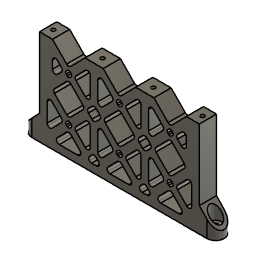
platform_hangfa-discovery-q2_top-plate-support-basic (Autodesk Fusion 360 design; units mm, degrees)
Autodesk Fusion 360 part; units mm, degrees
sketch "Sketch1" plane through (0, 0, 0) normal (0, 1, 0) x (1, 0, 0)
  circle A0 centre (0, 0) radius 2.25
  circle A1 centre (0, 0) radius 6
  circle A2 centre (0, 0) radius 9
  circle A3 centre (183.5, 0) radius 2.25
  circle A4 centre (183.5, 0) radius 6
  circle A5 centre (183.5, 0) radius 9
  line L0 (0, 0) -> (183.5, 0)
  line L1 (0, -9) -> (183.5, -9)
  line L2 (0, 9) -> (183.5, 9)
  line L3 (91.75, 9) -> (91.75, -9)
  line L4 (8, 9) -> (175.5, 9)
  line L5 (175.5, 9) -> (175.5, -9)
  line L6 (175.5, -9) -> (8, -9)
  line L7 (8, -9) -> (8, 9)
  line L8 (8, 9) -> (175.5, -9) construction
  line L9 (175.5, 9) -> (8, -9) construction
  line L10 (8, 9) -> (16, 9)
  line L11 (16, 9) -> (16, -9)
  line L12 (16, -9) -> (8, -9)
  line L13 (8, -9) -> (8, 9)
  line L14 (61.1667, -9) -> (61.1667, 9)
  line L15 (61.1667, 9) -> (69.1667, 9)
  line L16 (69.1667, 9) -> (69.1667, -9)
  line L17 (69.1667, -9) -> (61.1667, -9)
  line L18 (114.3333, -9) -> (114.3333, 9)
  line L19 (114.3333, 9) -> (122.3333, 9)
  line L20 (122.3333, 9) -> (122.3333, -9)
  line L21 (122.3333, -9) -> (114.3333, -9)
  line L22 (167.5, -9) -> (167.5, 9)
  line L23 (167.5, 9) -> (175.5, 9)
  line L24 (175.5, 9) -> (175.5, -9)
  line L25 (175.5, -9) -> (167.5, -9)
  point P0 (183.5, 0)
  point P1 (91.75, 0)
  dimension "d1" = 4.5
  dimension "d2" = 12
  dimension "d3" = 18
  dimension "d6" = 183.5
  dimension "d7" = 0
  dimension "d11" = 9
  dimension "d12" = -9
  dimension "d16" = 167.5
  dimension "d17" = 18
  dimension "d18" = 8
  dimension "d19" = 18
  dimension "d22" = 159.5
  dimension "d23" = 0
  constraint coincident A0.centre A1.centre
  constraint concentric A0 A1
  constraint coincident P0 A3.centre
  constraint midpoint L2 L3.start
  constraint midpoint L1 L3.end
  constraint perpendicular L1 L3
  constraint horizontal L4
  constraint perpendicular L4 L5
  constraint parallel L4 L6
  constraint parallel L5 L7
  constraint coincident L8 P1
  constraint coincident L9 P1
  constraint midpoint L3 P1
  constraint horizontal L10
  constraint vertical L11
  constraint horizontal L12
  constraint vertical L13
  measures "d1" diameter of A0
  measures "d2" diameter of A1
  measures "d3" diameter of A2
  measures "d16" distance of L5.end L6.end
  measures "d17" distance of L4.end L5.end
  measures "d18" distance of L4.start L10.end
  measures "d19" distance of L4.start L6.end
extrude "Extrude1" add sketch "Sketch1" against normal blind 8 contours A1 | A2 L7 L13 | A2 L2 L7 L13 | A2 L1 L7 L13 | A2 L0 L2 L4 L7 L10 L11 L13 | A2 L0 L7 L13 | A2 L0 L7 L13 | A2 L0 L1 L6 L7 L11 L12 L13 | L0 L2 L4 L11 L14 | L0 L1 L6 L11 L14 | L0 L2 L4 L14 L15 L16 | L0 L1 L6 L14 L16 L17 | L0 L2 L3 L4 L16 | L0 L1 L3 L6 L16 | L0 L2 L3 L4 L18 | L0 L1 L3 L6 L18 | L0 L2 L4 L18 L19 L20 | L0 L1 L6 L18 L20 L21 | L0 L2 L4 L20 L22 | L0 L1 L6 L20 L22 | A5 L0 L2 L4 L5 L22 L23 L24 | A5 L0 L1 L5 L6 L22 L24 L25 | A5 L2 L5 L24 | A5 L1 L5 L24 | A5 L0 L5 L24 | A5 L0 L5 L24 | A5 L5 L24 | A4
extrude "Extrude2" add sketch "Sketch1" along normal blind 92 contours A2 L0 L2 L4 L7 L10 L11 L13 | A2 L0 L7 L13 | A2 L0 L7 L13 | A2 L0 L1 L6 L7 L11 L12 L13 | L0 L2 L4 L14 L15 L16 | L0 L1 L6 L14 L16 L17 | L0 L2 L4 L18 L19 L20 | L0 L1 L6 L18 L20 L21 | A5 L0 L2 L4 L5 L22 L23 L24 | A5 L0 L1 L5 L6 L22 L24 L25 | A5 L0 L5 L24 | A5 L0 L5 L24
extrude "Extrude3" add sketch "Sketch1" along normal blind 18 contours A2 L7 L13 | A2 L2 L7 L13 | A2 L1 L7 L13 | A5 L2 L5 L24 | A5 L1 L5 L24 | A5 L5 L24
sketch "Sketch2" plane through (0, 0, 9) normal (0, 0, 1) x (1, 0, 0)
  line L0 (0, 18) -> (0, -8)
  line L1 (0, -8) -> (183.5, -8)
  line L2 (183.5, -8) -> (183.5, 18)
  line L3 (183.5, 18) -> (175.5, 18)
  line L4 (175.5, 18) -> (175.5, 92)
  line L5 (175.5, 92) -> (167.5, 92)
  line L6 (167.5, 92) -> (167.5, 0)
  line L7 (167.5, 0) -> (122.3333, 0)
  line L8 (122.3333, 0) -> (122.3333, 92)
  line L9 (122.3333, 92) -> (114.3333, 92)
  line L10 (114.3333, 92) -> (114.3333, 0)
  line L11 (114.3333, 0) -> (69.1667, 0)
  line L12 (69.1667, 0) -> (69.1667, 92)
  line L13 (69.1667, 92) -> (61.1667, 92)
  line L14 (61.1667, 92) -> (61.1667, 0)
  line L15 (61.1667, 0) -> (16, 0)
  line L16 (16, 0) -> (16, 92)
  line L17 (16, 92) -> (8, 92)
  line L18 (8, 92) -> (8, 18)
  line L19 (8, 18) -> (0, 18)
  line L20 (16, 0) -> (0, 0)
  line L21 (8, 18) -> (8, 0)
  line L22 (167.5, 0) -> (183.5, 0)
  line L23 (175.5, 18) -> (175.5, 0)
  line L24 (0, 0) -> (0, 18)
  line L25 (183.5, 0) -> (183.5, 18)
  line L26 (9, 0) -> (-9, 0)
  line L27 (-9, 0) -> (-9, 18)
  line L28 (-9, 18) -> (9, 18)
  line L29 (9, 18) -> (9, 0)
  line L30 (9, 0) -> (-9, 18) construction
  line L31 (-9, 0) -> (9, 18) construction
  line L32 (192.5, 0) -> (174.5, 0)
  line L33 (174.5, 0) -> (174.5, 18)
  line L34 (174.5, 18) -> (192.5, 18)
  line L35 (192.5, 18) -> (192.5, 0)
  line L36 (192.5, 0) -> (174.5, 18) construction
  line L37 (174.5, 0) -> (192.5, 18) construction
  line L38 (-9, 0) -> (8, 18)
  line L39 (192.5, 0) -> (175.5, 18)
  point P0 (0, 9)
  point P1 (183.5, 9)
  dimension "d32" = 18
  dimension "d33" = 18
  dimension "d34" = 18
  dimension "d35" = 18
  constraint coincident L15.end L16.start
  constraint coincident L20.end L24.start
  constraint coincident L18.end L19.start
  constraint midpoint L20 L21.end
  constraint coincident L6.end L7.start
  constraint coincident L2 L22.end
  constraint perpendicular L2 L22
  constraint coincident L3.end L4.start
  constraint midpoint L22 L23.end
  constraint coincident L0.start L19.end
  constraint coincident L2.end L3.start
  constraint horizontal L26
  constraint perpendicular L26 L27
  constraint parallel L26 L28
  constraint parallel L27 L29
  constraint coincident L30 P0
  constraint coincident L31 P0
  constraint midpoint L24 P0
  constraint horizontal L32
  constraint perpendicular L32 L33
  constraint parallel L32 L34
  constraint parallel L33 L35
  constraint coincident L36 P1
  constraint coincident L37 P1
  constraint midpoint L25 P1
  measures "d32" distance of L27.end L28.end
  measures "d33" distance of L26.end L27.end
  measures "d34" distance of L33.end L34.end
  measures "d35" distance of L32.end L33.end
extrude "Extrude4" cut sketch "Sketch2" against normal up to surface (18 mm away) contours L0 L24 L27 L28 L38 | L0 L19 L24 L28 L38 | L2 L3 L25 L34 L39 | L2 L25 L34 L35 L39
sketch "Sketch3" plane through (0, 0, 9) normal (0, 0, 1) x (1, 0, 0)
  line L0 (8, 18) -> (0, 9.5294)
  line L1 (0, 9.5294) -> (0, -8)
  line L2 (0, -8) -> (183.5, -8)
  line L3 (183.5, -8) -> (183.5, 9.5294)
  line L4 (183.5, 9.5294) -> (175.5, 18)
  line L5 (175.5, 18) -> (175.5, 92)
  line L6 (175.5, 92) -> (167.5, 92)
  line L7 (167.5, 92) -> (167.5, 0)
  line L8 (167.5, 0) -> (122.3333, 0)
  line L9 (122.3333, 0) -> (122.3333, 92)
  line L10 (122.3333, 92) -> (114.3333, 92)
  line L11 (114.3333, 92) -> (114.3333, 0)
  line L12 (114.3333, 0) -> (69.1667, 0)
  line L13 (69.1667, 0) -> (69.1667, 92)
  line L14 (69.1667, 92) -> (61.1667, 92)
  line L15 (61.1667, 92) -> (61.1667, 0)
  line L16 (61.1667, 0) -> (16, 0)
  line L17 (16, 0) -> (16, 92)
  line L18 (16, 92) -> (8, 92)
  line L19 (8, 92) -> (8, 18)
  line L20 (16, 0) -> (61.1667, 46)
  line L21 (61.1667, 46) -> (16, 92)
  line L22 (61.1667, 0) -> (16, 46)
  line L23 (16, 46) -> (61.1667, 92)
  line L24 (114.3333, 0) -> (69.1667, 46)
  line L25 (69.1667, 46) -> (114.3333, 92)
  line L26 (69.1667, 0) -> (114.3333, 46)
  line L27 (114.3333, 46) -> (69.1667, 92)
  line L28 (122.3333, 0) -> (167.5, 46)
  line L29 (167.5, 46) -> (122.3333, 92)
  line L30 (167.5, 0) -> (122.3333, 46)
  line L31 (122.3333, 46) -> (167.5, 92)
  line L32 (18.8542, -2.8025) -> (66.7725, 46)
  line L33 (66.7725, 46) -> (18.8542, 94.8025)
  line L34 (13.1458, 2.8025) -> (55.5608, 46)
  line L35 (55.5608, 46) -> (13.1458, 89.1975)
  line L36 (64.0208, 2.8025) -> (21.6058, 46)
  line L37 (21.6058, 46) -> (64.0208, 89.1975)
  line L38 (58.3125, -2.8025) -> (10.3942, 46)
  line L39 (10.3942, 46) -> (58.3125, 94.8025)
  line L40 (117.1875, 2.8025) -> (74.7725, 46)
  line L41 (74.7725, 46) -> (117.1875, 89.1975)
  line L42 (111.4792, -2.8025) -> (63.5608, 46)
  line L43 (63.5608, 46) -> (111.4792, 94.8025)
  line L44 (72.0208, -2.8025) -> (119.9392, 46)
  line L45 (119.9392, 46) -> (72.0208, 94.8025)
  line L46 (66.3125, 2.8025) -> (108.7275, 46)
  line L47 (108.7275, 46) -> (66.3125, 89.1975)
  line L48 (170.3542, 2.8025) -> (127.9392, 46)
  line L49 (127.9392, 46) -> (170.3542, 89.1975)
  line L50 (164.6458, -2.8025) -> (116.7275, 46)
  line L51 (116.7275, 46) -> (164.6458, 94.8025)
  line L52 (125.1875, -2.8025) -> (173.1058, 46)
  line L53 (173.1058, 46) -> (125.1875, 94.8025)
  line L54 (119.4792, 2.8025) -> (161.8942, 46)
  line L55 (161.8942, 46) -> (119.4792, 89.1975)
  line L56 (16, 92) -> (167.5, 92)
  dimension "d38" = 4
  dimension "d39" = -4
  dimension "d40" = 4
  dimension "d41" = -4
  dimension "d42" = 4
  dimension "d43" = -4
  dimension "d44" = 4
  dimension "d45" = -4
  dimension "d46" = 4
  dimension "d47" = -4
  dimension "d48" = 4
  dimension "d49" = -4
  constraint coincident L16.end L17.start
  constraint midpoint L15 L20.end
  constraint coincident L17.end L18.start
  constraint coincident L15.end L16.start
  constraint midpoint L17 L22.end
  constraint coincident L14.end L15.start
  constraint coincident L11.end L12.start
  constraint midpoint L13 L24.end
  constraint coincident L10.end L11.start
  constraint coincident L12.end L13.start
  constraint midpoint L11 L26.end
  constraint coincident L13.end L14.start
  constraint coincident L8.end L9.start
  constraint midpoint L7 L28.end
  constraint coincident L9.end L10.start
  constraint coincident L7.end L8.start
  constraint midpoint L9 L30.end
  constraint coincident L6.end L7.start
extrude "Extrude5" add sketch "Sketch3" against normal up to surface (18 mm away) contours L17 L21 L35 L39 | L21 L33 L39 L56 | L21 L23 L33 L39 | L21 L23 L35 L39 | L17 L23 L35 L39 | L21 L23 L33 L37 | L21 L23 L35 L37 | L23 L33 L39 L56 | L17 L22 L34 L38 | L22 L23 L34 L35 L36 L37 | L15 L21 L33 L37 | L20 L21 L34 L35 L36 L37 | L15 L23 L33 L37 | L20 L22 L34 L36 | L20 L22 L34 L38 | L15 L20 L32 L36 | L13 L27 L43 L47 | L27 L43 L45 L56 | L7 L31 L49 L53 | L31 L51 L53 L56 | L17 L20 L34 L38 | L20 L22 L32 L38 | L20 L22 L32 L36 | L25 L27 L43 L45 | L25 L27 L43 L47 | L29 L31 L49 L53 | L29 L31 L51 L53 | L16 L20 L32 L38 | L15 L22 L32 L36 | L16 L22 L32 L38 | L13 L25 L43 L47 | L25 L27 L41 L47 | L25 L27 L41 L45 | L25 L43 L45 L56 | L7 L29 L49 L53 | L29 L31 L51 L55 | L29 L31 L49 L55 | L29 L51 L53 L56 | L13 L24 L42 L46 | L24 L25 L40 L41 L46 L47 | L11 L25 L41 L45 | L11 L27 L41 L45 | L26 L27 L40 L41 L46 L47 | L7 L28 L48 L52 | L28 L29 L48 L49 L54 L55 | L9 L29 L51 L55 | L30 L31 L48 L49 L54 L55 | L9 L31 L51 L55 | L13 L26 L42 L46 | L24 L26 L42 L46 | L24 L26 L40 L46 | L11 L26 L40 L44 | L28 L30 L48 L52 | L28 L30 L48 L54 | L9 L30 L50 L54 | L12 L26 L42 L44 | L24 L26 L42 L44 | L24 L26 L40 L44 | L7 L30 L48 L52 | L28 L30 L50 L52 | L28 L30 L50 L54 | L12 L24 L42 L44 | L11 L24 L40 L44 | L8 L30 L50 L52 | L8 L28 L50 L52 | L9 L28 L50 L54
sketch "Sketch9" plane through (0, 0, 9) normal (0, 0, 1) x (1, 0, 0)
  line L0 (127.9392, 92) -> (108.7275, 92)
  line L1 (108.7275, 92) -> (91.75, 74.7093)
  line L2 (91.75, 74.7093) -> (74.7725, 92)
  line L3 (74.7725, 92) -> (55.5608, 92)
  line L4 (55.5608, 92) -> (38.5833, 74.7093)
  line L5 (38.5833, 74.7093) -> (21.6058, 92)
  line L6 (21.6058, 92) -> (8, 92)
  line L7 (8, 92) -> (8, 18)
  line L8 (8, 18) -> (0, 9.5294)
  line L9 (0, 9.5294) -> (0, -8)
  line L10 (0, -8) -> (183.5, -8)
  line L11 (183.5, -8) -> (183.5, 9.5294)
  line L12 (183.5, 9.5294) -> (175.5, 18)
  line L13 (175.5, 18) -> (175.5, 92)
  line L14 (175.5, 92) -> (161.8942, 92)
  line L15 (161.8942, 92) -> (144.9167, 74.7093)
  line L16 (144.9167, 74.7093) -> (127.9392, 92)
  line L17 (122.3333, 86.2907) -> (139.3108, 69)
  line L18 (139.3108, 69) -> (122.3333, 51.7093)
  line L19 (122.3333, 51.7093) -> (122.3333, 86.2907)
  line L20 (122.3333, 40.2907) -> (139.3108, 23)
  line L21 (139.3108, 23) -> (122.3333, 5.7093)
  line L22 (122.3333, 5.7093) -> (122.3333, 40.2907)
  line L23 (127.9392, 0) -> (144.9167, 17.2907)
  line L24 (144.9167, 17.2907) -> (161.8942, 0)
  line L25 (161.8942, 0) -> (127.9392, 0)
  line L26 (167.5, 5.7093) -> (150.5225, 23)
  line L27 (150.5225, 23) -> (167.5, 40.2907)
  line L28 (167.5, 40.2907) -> (167.5, 5.7093)
  line L29 (161.8942, 46) -> (144.9167, 28.7093)
  line L30 (144.9167, 28.7093) -> (127.9392, 46)
  line L31 (127.9392, 46) -> (144.9167, 63.2907)
  line L32 (144.9167, 63.2907) -> (161.8942, 46)
  line L33 (167.5, 51.7093) -> (150.5225, 69)
  line L34 (150.5225, 69) -> (167.5, 86.2907)
  line L35 (167.5, 86.2907) -> (167.5, 51.7093)
  line L36 (69.1667, 86.2907) -> (86.1442, 69)
  line L37 (86.1442, 69) -> (69.1667, 51.7093)
  line L38 (69.1667, 51.7093) -> (69.1667, 86.2907)
  line L39 (69.1667, 40.2907) -> (86.1442, 23)
  line L40 (86.1442, 23) -> (69.1667, 5.7093)
  line L41 (69.1667, 5.7093) -> (69.1667, 40.2907)
  line L42 (74.7725, 0) -> (91.75, 17.2907)
  line L43 (91.75, 17.2907) -> (108.7275, 0)
  line L44 (108.7275, 0) -> (74.7725, 0)
  line L45 (114.3333, 5.7093) -> (97.3558, 23)
  line L46 (97.3558, 23) -> (114.3333, 40.2907)
  line L47 (114.3333, 40.2907) -> (114.3333, 5.7093)
  line L48 (108.7275, 46) -> (91.75, 28.7093)
  line L49 (91.75, 28.7093) -> (74.7725, 46)
  line L50 (74.7725, 46) -> (91.75, 63.2907)
  line L51 (91.75, 63.2907) -> (108.7275, 46)
  line L52 (114.3333, 51.7093) -> (97.3558, 69)
  line L53 (97.3558, 69) -> (114.3333, 86.2907)
  line L54 (114.3333, 86.2907) -> (114.3333, 51.7093)
  line L55 (16, 86.2907) -> (32.9775, 69)
  line L56 (32.9775, 69) -> (16, 51.7093)
  line L57 (16, 51.7093) -> (16, 86.2907)
  line L58 (16, 40.2907) -> (32.9775, 23)
  line L59 (32.9775, 23) -> (16, 5.7093)
  line L60 (16, 5.7093) -> (16, 40.2907)
  line L61 (21.6058, 0) -> (38.5833, 17.2907)
  line L62 (38.5833, 17.2907) -> (55.5608, 0)
  line L63 (55.5608, 0) -> (21.6058, 0)
  line L64 (61.1667, 5.7093) -> (44.1892, 23)
  line L65 (44.1892, 23) -> (61.1667, 40.2907)
  line L66 (61.1667, 40.2907) -> (61.1667, 5.7093)
  line L67 (55.5608, 46) -> (38.5833, 28.7093)
  line L68 (38.5833, 28.7093) -> (21.6058, 46)
  line L69 (21.6058, 46) -> (38.5833, 63.2907)
  line L70 (38.5833, 63.2907) -> (55.5608, 46)
  line L71 (61.1667, 51.7093) -> (44.1892, 69)
  line L72 (44.1892, 69) -> (61.1667, 86.2907)
  line L73 (61.1667, 86.2907) -> (61.1667, 51.7093)
  line L74 (21.6058, 46) -> (8, 46)
  line L75 (8, 46) -> (8, 92)
  line L76 (8, 92) -> (21.6058, 92)
  line L77 (21.6058, 92) -> (21.6058, 46)
  line L78 (161.8942, 46) -> (175.5, 46)
  line L79 (175.5, 46) -> (175.5, 92)
  line L80 (175.5, 92) -> (161.8942, 92)
  line L81 (161.8942, 92) -> (161.8942, 46)
  constraint horizontal L74
  constraint vertical L75
  constraint horizontal L76
  constraint vertical L77
  constraint coincident L6.end L7.start
  constraint coincident L68.end L69.start
  constraint horizontal L78
  constraint vertical L79
  constraint horizontal L80
  constraint vertical L81
  constraint coincident L13.end L14.start
  constraint coincident L29.start L32.end
extrude "Extrude10" add sketch "Sketch9" against normal up to surface (18 mm away) contours L33 L34 L35 L81 | L55 L56 L57 L77
fillet "Fillet4" radius 3 60 edges at (32.9775, 69, 0) (32.9775, 23, 0) (55.5608, 0, 0) (55.5608, 46, 0) (86.1442, 23, 0) (86.1442, 69, 0) (108.7275, 46, 0) (108.7275, 0, 0) (161.8942, 0, 0) (161.8942, 46, 0) (139.3108, 69, 0) (139.3108, 23, 0) (21.6058, 0, 0) (74.7725, 0, 0) (127.9392, 0, 0) (21.6058, 46, 0) (74.7725, 46, 0) (127.9392, 46, 0) (150.5225, 23, 0) (97.3558, 23, 0) (44.1892, 23, 0) (44.1892, 69, 0) (97.3558, 69, 0) (150.5225, 69, 0) (91.75, 28.7093, 0) (38.5833, 28.7093, 0) (38.5833, 74.7093, 0) (91.75, 74.7093, 0) (144.9167, 74.7093, 0) (144.9167, 28.7093, 0) (16, 5.7093, 0) (21.6058, 57.4186, 0) (69.1667, 5.7093, 0) (69.1667, 51.7093, 0) (122.3333, 5.7093, 0) (122.3333, 51.7093, 0) (161.8942, 57.4186, 0) (167.5, 5.7093, 0) (114.3333, 51.7093, 0) (114.3333, 5.7093, 0) (61.1667, 51.7093, 0) (61.1667, 5.7093, 0) (61.1667, 86.2907, 0) (38.5833, 63.2907, 0) (61.1667, 40.2907, 0) (38.5833, 17.2907, 0) (114.3333, 86.2907, 0) (91.75, 63.2907, 0) (91.75, 17.2907, 0) (114.3333, 40.2907, 0) (161.8942, 80.5814, 0) (144.9167, 63.2907, 0) (144.9167, 17.2907, 0) (167.5, 40.2907, 0) (16, 40.2907, 0) (69.1667, 86.2907, 0) (122.3333, 86.2907, 0) (122.3333, 40.2907, 0) (69.1667, 40.2907, 0) (21.6058, 80.5814, 0)
sketch "Sketch10" plane through (0, 0, 9) normal (0, 0, 1) x (1, 0, 0)
  line L0 (127.9392, 92) -> (108.7275, 92)
  line L1 (108.7275, 92) -> (93.8906, 76.8894)
  arc A0 (89.6094, 76.8894) -> (93.8906, 76.8894) centre (91.75, 78.9912) ccw
  line L2 (89.6094, 76.8894) -> (74.7725, 92)
  line L3 (74.7725, 92) -> (55.5608, 92)
  line L4 (55.5608, 92) -> (40.724, 76.8894)
  arc A1 (36.4427, 76.8894) -> (40.724, 76.8894) centre (38.5833, 78.9912) ccw
  line L5 (36.4427, 76.8894) -> (21.6058, 92)
  line L6 (21.6058, 92) -> (8, 92)
  line L7 (8, 92) -> (8, 18)
  line L8 (8, 18) -> (0, 9.5294)
  line L9 (0, 9.5294) -> (0, -8)
  line L10 (0, -8) -> (183.5, -8)
  line L11 (183.5, -8) -> (183.5, 9.5294)
  line L12 (183.5, 9.5294) -> (175.5, 18)
  line L13 (175.5, 18) -> (175.5, 92)
  line L14 (175.5, 92) -> (161.8942, 92)
  line L15 (161.8942, 92) -> (147.0573, 76.8894)
  arc A2 (142.776, 76.8894) -> (147.0573, 76.8894) centre (144.9167, 78.9912) ccw
  line L16 (142.776, 76.8894) -> (127.9392, 92)
  line L17 (122.3333, 59.0466) -> (122.3333, 78.9534)
  arc A3 (127.474, 81.0553) -> (122.3333, 78.9534) centre (125.3333, 78.9534) ccw
  line L18 (127.474, 81.0553) -> (137.2471, 71.1018)
  arc A4 (137.2471, 66.8982) -> (137.2471, 71.1018) centre (135.1064, 69) ccw
  line L19 (137.2471, 66.8982) -> (127.474, 56.9447)
  arc A5 (122.3333, 59.0466) -> (127.474, 56.9447) centre (125.3333, 59.0466) ccw
  line L20 (122.3333, 13.0466) -> (122.3333, 32.9534)
  arc A6 (127.474, 35.0553) -> (122.3333, 32.9534) centre (125.3333, 32.9534) ccw
  line L21 (127.474, 35.0553) -> (137.2471, 25.1018)
  arc A7 (137.2471, 20.8982) -> (137.2471, 25.1018) centre (135.1064, 23) ccw
  line L22 (137.2471, 20.8982) -> (127.474, 10.9447)
  arc A8 (122.3333, 13.0466) -> (127.474, 10.9447) centre (125.3333, 13.0466) ccw
  line L23 (132.9486, 5.1018) -> (142.776, 15.1106)
  arc A9 (147.0573, 15.1106) -> (142.776, 15.1106) centre (144.9167, 13.0088) ccw
  line L24 (147.0573, 15.1106) -> (156.8847, 5.1018)
  arc A10 (154.7441, 0) -> (156.8847, 5.1018) centre (154.7441, 3) ccw
  line L25 (154.7441, 0) -> (135.0892, 0)
  arc A11 (132.9486, 5.1018) -> (135.0892, 0) centre (135.0892, 3) ccw
  line L26 (162.3594, 10.9447) -> (152.5863, 20.8982)
  arc A12 (152.5863, 25.1018) -> (152.5863, 20.8982) centre (154.7269, 23) ccw
  line L27 (152.5863, 25.1018) -> (162.3594, 35.0553)
  arc A13 (167.5, 32.9534) -> (162.3594, 35.0553) centre (164.5, 32.9534) ccw
  line L28 (167.5, 32.9534) -> (167.5, 13.0466)
  arc A14 (162.3594, 10.9447) -> (167.5, 13.0466) centre (164.5, 13.0466) ccw
  line L29 (159.8304, 43.8982) -> (147.0573, 30.8894)
  arc A15 (142.776, 30.8894) -> (147.0573, 30.8894) centre (144.9167, 32.9912) ccw
  line L30 (142.776, 30.8894) -> (130.0029, 43.8982)
  arc A16 (130.0029, 48.1018) -> (130.0029, 43.8982) centre (132.1436, 46) ccw
  line L31 (130.0029, 48.1018) -> (142.776, 61.1106)
  arc A17 (147.0573, 61.1106) -> (142.776, 61.1106) centre (144.9167, 59.0088) ccw
  line L32 (147.0573, 61.1106) -> (159.8304, 48.1018)
  arc A18 (159.8304, 43.8982) -> (159.8304, 48.1018) centre (157.6898, 46) ccw
  line L33 (156.7535, 62.654) -> (152.5863, 66.8982)
  arc A19 (152.5863, 71.1018) -> (152.5863, 66.8982) centre (154.7269, 69) ccw
  line L34 (152.5863, 71.1018) -> (156.7535, 75.346)
  arc A20 (161.8942, 73.2441) -> (156.7535, 75.346) centre (158.8942, 73.2441) ccw
  line L35 (161.8942, 73.2441) -> (161.8942, 64.7559)
  arc A21 (156.7535, 62.654) -> (161.8942, 64.7559) centre (158.8942, 64.7559) ccw
  line L36 (69.1667, 59.0466) -> (69.1667, 78.9534)
  arc A22 (74.3073, 81.0553) -> (69.1667, 78.9534) centre (72.1667, 78.9534) ccw
  line L37 (74.3073, 81.0553) -> (84.0804, 71.1018)
  arc A23 (84.0804, 66.8982) -> (84.0804, 71.1018) centre (81.9398, 69) ccw
  line L38 (84.0804, 66.8982) -> (74.3073, 56.9447)
  arc A24 (69.1667, 59.0466) -> (74.3073, 56.9447) centre (72.1667, 59.0466) ccw
  line L39 (69.1667, 13.0466) -> (69.1667, 32.9534)
  arc A25 (74.3073, 35.0553) -> (69.1667, 32.9534) centre (72.1667, 32.9534) ccw
  line L40 (74.3073, 35.0553) -> (84.0804, 25.1018)
  arc A26 (84.0804, 20.8982) -> (84.0804, 25.1018) centre (81.9398, 23) ccw
  line L41 (84.0804, 20.8982) -> (74.3073, 10.9447)
  arc A27 (69.1667, 13.0466) -> (74.3073, 10.9447) centre (72.1667, 13.0466) ccw
  line L42 (79.7819, 5.1018) -> (89.6094, 15.1106)
  arc A28 (93.8906, 15.1106) -> (89.6094, 15.1106) centre (91.75, 13.0088) ccw
  line L43 (93.8906, 15.1106) -> (103.7181, 5.1018)
  arc A29 (101.5774, 0) -> (103.7181, 5.1018) centre (101.5774, 3) ccw
  line L44 (101.5774, 0) -> (81.9226, 0)
  arc A30 (79.7819, 5.1018) -> (81.9226, 0) centre (81.9226, 3) ccw
  line L45 (109.1927, 10.9447) -> (99.4196, 20.8982)
  arc A31 (99.4196, 25.1018) -> (99.4196, 20.8982) centre (101.5602, 23) ccw
  line L46 (99.4196, 25.1018) -> (109.1927, 35.0553)
  arc A32 (114.3333, 32.9534) -> (109.1927, 35.0553) centre (111.3333, 32.9534) ccw
  line L47 (114.3333, 32.9534) -> (114.3333, 13.0466)
  arc A33 (109.1927, 10.9447) -> (114.3333, 13.0466) centre (111.3333, 13.0466) ccw
  line L48 (106.6637, 43.8982) -> (93.8906, 30.8894)
  arc A34 (89.6094, 30.8894) -> (93.8906, 30.8894) centre (91.75, 32.9912) ccw
  line L49 (89.6094, 30.8894) -> (76.8363, 43.8982)
  arc A35 (76.8363, 48.1018) -> (76.8363, 43.8982) centre (78.9769, 46) ccw
  line L50 (76.8363, 48.1018) -> (89.6094, 61.1106)
  arc A36 (93.8906, 61.1106) -> (89.6094, 61.1106) centre (91.75, 59.0088) ccw
  line L51 (93.8906, 61.1106) -> (106.6637, 48.1018)
  arc A37 (106.6637, 43.8982) -> (106.6637, 48.1018) centre (104.5231, 46) ccw
  line L52 (109.1927, 56.9447) -> (99.4196, 66.8982)
  arc A38 (99.4196, 71.1018) -> (99.4196, 66.8982) centre (101.5602, 69) ccw
  line L53 (99.4196, 71.1018) -> (109.1927, 81.0553)
  arc A39 (114.3333, 78.9534) -> (109.1927, 81.0553) centre (111.3333, 78.9534) ccw
  line L54 (114.3333, 78.9534) -> (114.3333, 59.0466)
  arc A40 (109.1927, 56.9447) -> (114.3333, 59.0466) centre (111.3333, 59.0466) ccw
  arc A41 (21.6058, 64.7559) -> (26.7465, 62.654) centre (24.6058, 64.7559) ccw
  line L55 (21.6058, 64.7559) -> (21.6058, 73.2441)
  arc A42 (26.7465, 75.346) -> (21.6058, 73.2441) centre (24.6058, 73.2441) ccw
  line L56 (26.7465, 75.346) -> (30.9137, 71.1018)
  arc A43 (30.9137, 66.8982) -> (30.9137, 71.1018) centre (28.7731, 69) ccw
  line L57 (30.9137, 66.8982) -> (26.7465, 62.654)
  line L58 (16, 13.0466) -> (16, 32.9534)
  arc A44 (21.1406, 35.0553) -> (16, 32.9534) centre (19, 32.9534) ccw
  line L59 (21.1406, 35.0553) -> (30.9137, 25.1018)
  arc A45 (30.9137, 20.8982) -> (30.9137, 25.1018) centre (28.7731, 23) ccw
  line L60 (30.9137, 20.8982) -> (21.1406, 10.9447)
  arc A46 (16, 13.0466) -> (21.1406, 10.9447) centre (19, 13.0466) ccw
  line L61 (26.6153, 5.1018) -> (36.4427, 15.1106)
  arc A47 (40.724, 15.1106) -> (36.4427, 15.1106) centre (38.5833, 13.0088) ccw
  line L62 (40.724, 15.1106) -> (50.5514, 5.1018)
  arc A48 (48.4108, 0) -> (50.5514, 5.1018) centre (48.4108, 3) ccw
  line L63 (48.4108, 0) -> (28.7559, 0)
  arc A49 (26.6153, 5.1018) -> (28.7559, 0) centre (28.7559, 3) ccw
  line L64 (56.026, 10.9447) -> (46.2529, 20.8982)
  arc A50 (46.2529, 25.1018) -> (46.2529, 20.8982) centre (48.3936, 23) ccw
  line L65 (46.2529, 25.1018) -> (56.026, 35.0553)
  arc A51 (61.1667, 32.9534) -> (56.026, 35.0553) centre (58.1667, 32.9534) ccw
  line L66 (61.1667, 32.9534) -> (61.1667, 13.0466)
  arc A52 (56.026, 10.9447) -> (61.1667, 13.0466) centre (58.1667, 13.0466) ccw
  line L67 (53.4971, 43.8982) -> (40.724, 30.8894)
  arc A53 (36.4427, 30.8894) -> (40.724, 30.8894) centre (38.5833, 32.9912) ccw
  line L68 (36.4427, 30.8894) -> (23.6696, 43.8982)
  arc A54 (23.6696, 48.1018) -> (23.6696, 43.8982) centre (25.8102, 46) ccw
  line L69 (23.6696, 48.1018) -> (36.4427, 61.1106)
  arc A55 (40.724, 61.1106) -> (36.4427, 61.1106) centre (38.5833, 59.0088) ccw
  line L70 (40.724, 61.1106) -> (53.4971, 48.1018)
  arc A56 (53.4971, 43.8982) -> (53.4971, 48.1018) centre (51.3564, 46) ccw
  line L71 (56.026, 56.9447) -> (46.2529, 66.8982)
  arc A57 (46.2529, 71.1018) -> (46.2529, 66.8982) centre (48.3936, 69) ccw
  line L72 (46.2529, 71.1018) -> (56.026, 81.0553)
  arc A58 (61.1667, 78.9534) -> (56.026, 81.0553) centre (58.1667, 78.9534) ccw
  line L73 (61.1667, 78.9534) -> (61.1667, 59.0466)
  arc A59 (56.026, 56.9447) -> (61.1667, 59.0466) centre (58.1667, 59.0466) ccw
  line L74 (54.3564, 46) -> (75.9769, 46)
  line L75 (107.5231, 46) -> (129.1436, 46)
  line L76 (104.3438, 1.8393) -> (132.3229, 1.8393)
  line L77 (51.1771, 1.8393) -> (79.1562, 1.8393)
  line L78 (73.1667, 46) -> (65.1667, 54)
  line L79 (65.1667, 54) -> (57.1667, 46)
  line L80 (57.1667, 46) -> (65.1667, 38)
  line L81 (65.1667, 38) -> (73.1667, 46)
  line L82 (110.3333, 46) -> (118.3333, 38)
  line L83 (118.3333, 38) -> (126.3333, 46)
  line L84 (126.3333, 46) -> (118.3333, 54)
  line L85 (118.3333, 54) -> (110.3333, 46)
  line L86 (57.1667, 1.8393) -> (65.1667, -6.1607)
  line L87 (65.1667, -6.1607) -> (73.1667, 1.8393)
  line L88 (73.1667, 1.8393) -> (65.1667, 9.8393)
  line L89 (65.1667, 9.8393) -> (57.1667, 1.8393)
  line L90 (110.3333, 1.8393) -> (118.3333, -6.1607)
  line L91 (118.3333, -6.1607) -> (126.3333, 1.8393)
  line L92 (126.3333, 1.8393) -> (118.3333, 9.8393)
  line L93 (118.3333, 9.8393) -> (110.3333, 1.8393)
  line L94 (48.4108, 0) -> (135.0892, 0)
  line L95 (57.1667, 1.8393) -> (55.3274, 0)
  line L96 (73.1667, 1.8393) -> (75.006, 0)
  line L97 (110.3333, 1.8393) -> (108.494, 0)
  line L98 (126.3333, 1.8393) -> (128.1726, 0)
  line L99 (31.7731, 23) -> (45.3936, 23)
  line L100 (31.7731, 69) -> (45.3936, 69)
  line L101 (84.9398, 69) -> (98.5602, 69)
  line L102 (84.9398, 23) -> (98.5602, 23)
  line L103 (138.1064, 23) -> (151.7269, 23)
  line L104 (138.1064, 69) -> (151.7269, 69)
  line L105 (34.5833, 69) -> (38.5833, 65)
  line L106 (38.5833, 65) -> (42.5833, 69)
  line L107 (42.5833, 69) -> (38.5833, 73)
  line L108 (38.5833, 73) -> (34.5833, 69)
  line L109 (34.5833, 23) -> (38.5833, 19)
  line L110 (38.5833, 19) -> (42.5833, 23)
  line L111 (42.5833, 23) -> (38.5833, 27)
  line L112 (38.5833, 27) -> (34.5833, 23)
  line L113 (87.75, 23) -> (91.75, 19)
  line L114 (91.75, 19) -> (95.75, 23)
  line L115 (95.75, 23) -> (91.75, 27)
  line L116 (91.75, 27) -> (87.75, 23)
  line L117 (87.75, 69) -> (91.75, 65)
  line L118 (91.75, 65) -> (95.75, 69)
  line L119 (95.75, 69) -> (91.75, 73)
  line L120 (91.75, 73) -> (87.75, 69)
  line L121 (140.9167, 69) -> (144.9167, 65)
  line L122 (144.9167, 65) -> (148.9167, 69)
  line L123 (148.9167, 69) -> (144.9167, 73)
  line L124 (144.9167, 73) -> (140.9167, 69)
  line L125 (140.9167, 23) -> (144.9167, 19)
  line L126 (144.9167, 19) -> (148.9167, 23)
  line L127 (148.9167, 23) -> (144.9167, 27)
  line L128 (144.9167, 27) -> (140.9167, 23)
  point P0 (65.1667, 46)
  point P1 (118.3333, 46)
  point P2 (65.1667, 1.8393)
  point P3 (118.3333, 1.8393)
  point P4 (38.5833, 69)
  point P5 (38.5833, 23)
  point P6 (91.75, 23)
  point P7 (91.75, 69)
  point P8 (144.9167, 69)
  point P9 (144.9167, 23)
  dimension "d78" = 8
  dimension "d79" = 8
  dimension "d80" = 8
  dimension "d81" = 8
  dimension "d86" = 4
  dimension "d87" = 4
  dimension "d88" = 4
  dimension "d89" = 4
  dimension "d90" = 4
  dimension "d91" = 4
  constraint midpoint A56 L74.start
  constraint midpoint A35 L74.end
  constraint midpoint A37 L75.start
  constraint midpoint A16 L75.end
  constraint midpoint A29 L76.start
  constraint midpoint A11 L76.end
  constraint midpoint A48 L77.start
  constraint midpoint A30 L77.end
  constraint midpoint L74 P0
  constraint midpoint L75 P1
  constraint midpoint L77 P2
  constraint midpoint L76 P3
  constraint coincident A48.start L63.start
  constraint coincident L25.end A11.end
  constraint coincident L94 L95.end
  constraint perpendicular L86 L95
  constraint coincident L94 L96.end
  constraint perpendicular L95 L96
  constraint coincident L94 L97.end
  constraint perpendicular L96 L97
  constraint coincident L94 L98.end
  constraint perpendicular L91 L98
  constraint midpoint A45 L99.start
  constraint midpoint A50 L99.end
  constraint midpoint A43 L100.start
  constraint midpoint A57 L100.end
  constraint midpoint A23 L101.start
  constraint midpoint A38 L101.end
  constraint midpoint A26 L102.start
  constraint midpoint A31 L102.end
  constraint midpoint A7 L103.start
  constraint midpoint A12 L103.end
  constraint midpoint A4 L104.start
  constraint midpoint A19 L104.end
  constraint midpoint L100 P4
  constraint coincident L99 L109.start
  constraint midpoint L99 P5
  constraint midpoint L102 P6
  constraint midpoint L101 P7
  constraint midpoint L104 P8
  constraint midpoint L103 P9
  measures "d78" distance of L78.start P0
  measures "d79" distance of L82.start P1
  measures "d80" distance of L86.start P2
  measures "d81" distance of L90.start P3
  measures "d86" distance of L105.start P4
  measures "d87" distance of L109.start P5
  measures "d88" distance of L113.start P6
  measures "d89" distance of L117.start P7
  measures "d90" distance of L121.start P8
  measures "d91" distance of L125.start P9
extrude "Extrude11" cut sketch "Sketch10" against normal up to surface (18 mm away) contours L76 L90 L91 L94 | L91 L94 L98 | L76 L92 L93 | L90 L94 L97 | L87 L94 L96 | L77 L86 L87 L94 | L77 L88 L89 | L86 L94 L95 | L74 L78 L79 | L74 L80 L81 | L75 L84 L85 | L75 L82 L83
fillet "Fillet5" radius 3 14 edges at (126.3333, 46, 0) (118.3333, 54, 0) (110.3333, 46, 0) (57.1667, 46, 0) (55.3274, 0, 0) (108.494, 0, 0) (75.006, 0, 0) (73.1667, 46, 0) (128.1726, 0, 0) (65.1667, 38, 0) (118.3333, 38, 0) (65.1667, 54, 0) (118.3333, 9.8393, 0) (65.1667, 9.8393, 0)
extrude "Extrude12" cut sketch "Sketch10" against normal up to surface (18 mm away) contours L99 L111 L112 | L99 L109 L110 | L100 L107 L108 | L100 L105 L106 | L101 L119 L120 | L101 L117 L118 | L102 L115 L116 | L102 L113 L114 | L103 L127 L128 | L103 L125 L126 | L104 L123 L124 | L104 L121 L122
fillet "Fillet6" radius 2 24 edges at (38.5833, 65, 0) (38.5833, 19, 0) (91.75, 19, 0) (91.75, 65, 0) (144.9167, 65, 0) (144.9167, 19, 0) (140.9167, 69, 0) (140.9167, 23, 0) (87.75, 23, 0) (34.5833, 23, 0) (34.5833, 69, 0) (148.9167, 69, 0) (148.9167, 23, 0) (95.75, 23, 0) (95.75, 69, 0) (42.5833, 69, 0) (42.5833, 23, 0) (87.75, 69, 0) (38.5833, 73, 0) (38.5833, 27, 0) (91.75, 73, 0) (91.75, 27, 0) (144.9167, 27, 0) (144.9167, 73, 0)
sketch "Sketch11" plane through (0, 92, 0) normal (0, 1, 0) x (-1, 0, 0)
  line L0 (-8, 9) -> (-21.6058, 9)
  line L1 (-21.6058, 9) -> (-21.6058, -9)
  line L2 (-21.6058, -9) -> (-8, -9)
  line L3 (-8, -9) -> (-8, 9)
  line L4 (-8, 9) -> (-19.13, 9)
  line L5 (-19.13, 9) -> (-19.13, -9)
  line L6 (-19.13, -9) -> (-8, -9)
  line L7 (-8, -9) -> (-8, 9)
  line L8 (-8, 9) -> (-19.13, -9)
  circle A0 centre (-13.565, 0) radius 2
  dimension "d108" = 11.13
  dimension "d109" = 18
  dimension "d110" = 4
  constraint horizontal L4
  constraint vertical L5
  constraint horizontal L6
  constraint vertical L7
  constraint coincident L0.start L3.end
  constraint midpoint L8 A0.centre
  measures "d108" distance of L0.start L4.end
  measures "d109" distance of L0.start L2.end
  measures "d110" diameter of A0
extrude "Extrude13" cut sketch "Sketch11" against normal blind 20 contours L8 A0 | L8 A0
sketch "Sketch12" plane through (0, 92, 0) normal (0, 1, 0) x (-1, 0, 0)
  line L0 (-175.5, 9) -> (-175.5, -9)
  line L1 (-175.5, -9) -> (-161.8942, -9)
  line L2 (-161.8942, -9) -> (-161.8942, 9)
  line L3 (-161.8942, 9) -> (-175.5, 9)
  line L4 (-175.5, 9) -> (-164.37, 9)
  line L5 (-164.37, 9) -> (-164.37, -9)
  line L6 (-164.37, -9) -> (-175.5, -9)
  line L7 (-175.5, -9) -> (-175.5, 9)
  line L8 (-164.37, -9) -> (-175.5, 9)
  circle A0 centre (-169.935, 0) radius 2
  dimension "d113" = 11.13
  dimension "d114" = 18
  dimension "d115" = 4
  constraint horizontal L4
  constraint vertical L5
  constraint horizontal L6
  constraint vertical L7
  constraint coincident L0.start L3.end
  constraint midpoint L8 A0.centre
  measures "d113" distance of L0.start L4.end
  measures "d114" distance of L0.start L0.end
  measures "d115" diameter of A0
extrude "Extrude14" cut sketch "Sketch12" against normal blind 20 contours L8 A0 | L8 A0
hole "Hole5" at (65.1667, 92, 0) direction (0, -1, 0) diameter 4 depth 20 tip angle 180
hole "Hole6" at (118.3333, 92, 0) direction (0, -1, 0) diameter 4 depth 20 tip angle 180
equation "d1 = base2supp_screw_hole"
equation "d2 = base2supp_screw_head"
equation "d3 = base2supp_screw_outer"
equation "base2supp_screw_hole = 4.5 mm"
equation "base2supp_screw_head = 12 mm"
equation "base2supp_screw_outer = 18 mm"
equation "d11 = base2supp_screw_outer / 2"
equation "d12 = -base2supp_screw_outer / 2"
equation "supp_wall_thickness = 8 mm"
equation "supp_wall_outer_width = 167.5 mm"
equation "d16 = supp_wall_outer_width"
equation "d18 = supp_wall_thickness"
equation "d19 = base2supp_screw_outer"
equation "d22 = supp_wall_outer_width - supp_wall_thickness"
equation "base2supp_height = 8 mm"
equation "d25 = -base2supp_height"
equation "supp_height = 100 mm"
equation "d28 = supp_height - base2supp_height"
equation "d30 = base2supp_screw_outer"
equation "d32 = base2supp_screw_outer"
equation "d33 = base2supp_screw_outer"
equation "d34 = base2supp_screw_outer"
equation "d35 = base2supp_screw_outer"
equation "d38 = supp_wall_thickness / 2"
equation "d39 = -supp_wall_thickness / 2"
equation "d40 = supp_wall_thickness / 2"
equation "d41 = -supp_wall_thickness / 2"
equation "d42 = supp_wall_thickness / 2"
equation "d43 = -supp_wall_thickness / 2"
equation "d44 = supp_wall_thickness / 2"
equation "d45 = -supp_wall_thickness / 2"
equation "d46 = supp_wall_thickness / 2"
equation "d47 = -supp_wall_thickness / 2"
equation "d48 = supp_wall_thickness / 2"
equation "d49 = -supp_wall_thickness / 2"
equation "fence_fillet = 3 mm"
equation "plate2supp_screw_hole = 4 mm"
equation "d77 = fence_fillet"
equation "d78 = supp_wall_thickness"
equation "d79 = supp_wall_thickness"
equation "d80 = supp_wall_thickness"
equation "d81 = supp_wall_thickness"
equation "d85 = fence_fillet"
equation "d86 = supp_wall_thickness / 2"
equation "d87 = supp_wall_thickness / 2"
equation "d88 = supp_wall_thickness / 2"
equation "d89 = supp_wall_thickness / 2"
equation "d90 = supp_wall_thickness / 2"
equation "d91 = supp_wall_thickness / 2"
equation "d109 = base2supp_screw_outer"
equation "d110 = plate2supp_screw_hole"
equation "d114 = base2supp_screw_outer"
equation "d115 = plate2supp_screw_hole"
equation "d119 = plate2supp_screw_hole"
equation "d122 = plate2supp_screw_hole"
